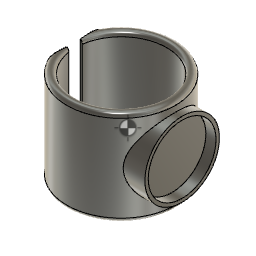
MagnetGlass:ring_plane (Autodesk Fusion 360 design; units mm, degrees)
Autodesk Fusion 360 part; units mm, degrees
sketch "スケッチ4" plane through (0, 0, 0) normal (0, 0, 1) x (1, 0, 0) in component "指輪"
  arc A0 (-6.9712, -3.9246) -> (-6.9712, 3.9246) centre (0, 0) ccw
  line L0 (-6.9712, 0.9595) -> (-0.9758, 0.9595)
  line L1 (-0.9758, 0.9595) -> (-0.9758, -1.0395)
  line L2 (-0.9758, -1.0395) -> (-6.9712, -1.0395)
  line L3 (-6.9712, 3.9246) -> (-6.9712, 0.9595)
  line L4 (-6.9712, -1.0395) -> (-6.9712, -3.9246)
  dimension "d29" = 16
  constraint coincident A0.centre origin
  constraint vertical L3
  constraint horizontal L0
  constraint vertical L1
  constraint horizontal L2
  constraint collinear L3 L4
  measures "d29" diameter of A0
extrude "押し出し1" add sketch "スケッチ4" along normal blind 14 makes body 1 in component "指輪"
cylinder "円柱プリミティブ1" add diameter 11 height 6 placed x (0, 0, -1) y (0, 1, 0) z (1, 0, 0) at (0, 23.0583, 6.8926) separate body makes body 2
move_body "移動1" bodies 2 to x (1, 0, 0) y (0, 1, 0) z (0, 0, 1) at (0, -23.0583, -6.8926)
move_body "移動2" bodies 2 to x (1, 0, 0) y (0, 1, 0) z (0, 0, 1) at (3, 0, 7)
combine "結合2" operation add target body 1 tool bodies 2 in component "指輪"
hole "穴4" at (0, 0, 14) direction (0, 0, -1) diameter 13.5 depth 15 tip angle 180 bodies 1 in component "指輪"
hole "穴6" at (9, 0, 7) direction (-1, 0, 0) diameter 10 depth 1.5 tip angle 180 bodies 1 in component "指輪"
fillet "フィレット4" radius 0.625 4 edges at (8, 0, 14) (6.7499, 0.0404, 14) (8, 0, 0) (6.7499, 0.0404, 0) on bodies 1 in component "指輪"
component "指輪" placed x (1, 0, 0) y (0, 1, 0) z (0, 0, 1) at (0, 0, 0)
